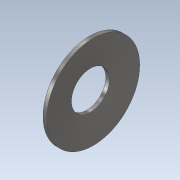
# Autodesk Inventor part: Tellerfeder_20_8
Saved by Autodesk Inventor 2021.4 (Build 254397000, 397)
## iProperties
Created: 2022-07-13
Part Number: Tellerfeder_20_8
Material: Stainless Steel
Document SubType Name: Modeling
Designer: alexw
Density: 8 g/cm^3
Appearance: Semi-Polished
Tellerfeder_Height: 1,400 mm
Author: alexw
Autodesk Inventor part; units mm, degrees
ref_plane "YZ Plane" through (0, 0, 0) normal (1, 0, 0) x (0, 1, 0)
ref_plane "XZ Plane" through (0, 0, 0) normal (0, 1, 0) x (-1, 0, 0)
ref_plane "XY Plane" through (0, 0, 0) normal (0, 0, 1) x (1, 0, 0)
sketch "Sketch1" plane through (0, 0, 0) normal (0, 0, 1) x (1, 0, 0)
  line L0 (0, 0) -> (1.4, 0) construction
  line L1 (0, 4.1) -> (0.5959, 10)
  line L2 (0.5959, 10) -> (1.4, 10)
  line L3 (1.4, 10) -> (0.8041, 4.1)
  line L4 (0.8041, 4.1) -> (0, 4.1)
  line L5 (0, -4.1) -> (0.5959, -10) construction
  line L6 (0.5959, -10) -> (1.4, -10) construction
  line L7 (1.4, -10) -> (0.8041, -4.1) construction
  line L8 (0.8041, -4.1) -> (0, -4.1) construction
  line L9 (0, 4.1) -> (0, -4.1) construction
  line L10 (1.4, 10) -> (1.4, -10) construction
  dimension "d0" = 20
  dimension "d1" = 8.2
  dimension "d2" = 0.8
  dimension "Tellerfeder_Height" = 1.4
  constraints: 22 end point, 4 symmetric about line, 2 horizontal, 2 midpoint, 2 parallel, 2 vertical
  measures "d0" diameter of L2 L0
  measures "d1" diameter of L4 L0
  measures "d2" distance between parallel lines of L3 L1
  measures "Tellerfeder_Height" horizontal distance of L1.start L2.end
revolve "Revolution1" add sketch "Sketch1" angle 360 about axis through (0, 0, 0) along (1, 0, 0)
body "Solid1"
